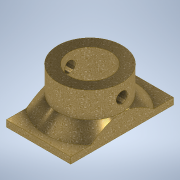
# Autodesk Inventor part: Union_Tubo_Soporte_Balancin
Saved by Autodesk Inventor 2022 (Build 260153000, 153)
## iProperties
Created: 2022-02-04
Part Number: Union_Tubo_Soporte_Balancin
Material: Generic
Document SubType Name: Modeling
Designer: hurta
Density: 1 g/cm^3
Appearance: Foil Gold
Author: hurta
Autodesk Inventor part; units mm, degrees
ref_plane "YZ Plane" through (0, 0, 0) normal (1, 0, 0) x (0, 1, 0)
ref_plane "XZ Plane" through (0, 0, 0) normal (0, 1, 0) x (-1, 0, 0)
ref_plane "XY Plane" through (0, 0, 0) normal (0, 0, 1) x (1, 0, 0)
sketch "Sketch1" plane through (0, 0, 0) normal (0, 1, 0) x (-1, 0, 0)
  circle A0 centre (0, 0) radius 16.15
  circle A1 centre (0, 0) radius 25
  dimension "d0" = 32.3
  dimension "d1" = 50
  constraints: 2 centre point, 2 coincident
  measures "d0" diameter of A0
  measures "d1" diameter of A1
extrude "Extrusion1" add sketch "Sketch1" along normal blind 30
sketch "Sketch2" plane through (0, 0, 0) normal (0, -1, 0) x (1, 0, 0)
  line L0 (25, -40) -> (-25, -40)
  line L1 (-25, -40) -> (-25, 40)
  line L2 (-25, 40) -> (25, 40)
  line L3 (25, 40) -> (25, -40)
  line L4 (25, -40) -> (-25, 40) construction
  line L5 (-25, -40) -> (25, 40) construction
  point P0 (0, 0)
  dimension "d4" = 80
  dimension "d5" = 50
  constraints: 12 end point, 2 midpoint, 2 parallel, 1 horizontal, 1 perpendicular
  measures "d4" distance of L2.end L0.start
  measures "d5" distance of L0.start L0.end
extrude "Extrusion2" add sketch "Sketch2" along normal blind 5
chamfer "Chamfer1" distance 10 angle 45 2 edges at (0, 0, 25) (0, 0, -25)
sketch "Sketch3" plane through (0, -5, 0) normal (0, -1, 0) x (1, 0, 0)
  line L0 (-25, 40) -> (-25, -40) projected
  line L1 (25, -40) -> (25, 40) projected
  point P0 (0, 0)
  point P1 (-5, 0)
  point P2 (5, 0)
  dimension "d11" = 20
  dimension "d12" = 20
  constraints: 2 horizontal alignment
  measures "d11" distance from line of L0 point (-5, 0)
  measures "d12" distance from line of L1 point (5, 0)
hole "Hole1" at (-5, -5, 0) at (5, -5, 0) direction (0, 1, 0) diameter 5.5 end through all clearance for "Hex Head Bolt" size "M5" standard "Ansi Metric M Profile"
sketch "Sketch4" plane through (-25, -5, -40) normal (-1, 0, 0) x (0, 0, 1)
  line L0 (65, 35) -> (15, 35) projected
  point P0 (40, 5)
  point P1 (40, 25)
  dimension "d20" = 10
  constraints: 1 vertical alignment
  measures "d20" distance from line of point (40, 25) L0
hole "Hole2" at (-25, 20, 0) direction (1, 0, 0) diameter 8.5 end through all clearance for "Hex Head Bolt" size "M8" standard "Ansi Metric M Profile"
equation "\"d12\" = d11"
body "Solid1"
